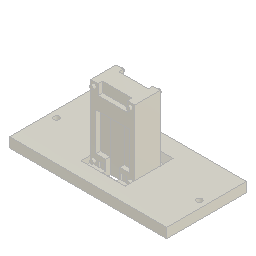
Nabu-SD-Backplate (Autodesk Fusion 360 design; units mm, degrees)
Autodesk Fusion 360 part; units mm, degrees
sketch "Sketch1" plane through (0, 0, 0) normal (0, 0, 1) x (1, 0, 0)
  line L0 (-42.75, -21.675) -> (42.75, -21.675)
  line L1 (42.75, -21.675) -> (42.75, 21.675)
  line L2 (42.75, 21.675) -> (-42.75, 21.675)
  line L3 (-42.75, 21.675) -> (-42.75, -21.675)
  line L4 (-35.5, -20) -> (35.5, -20)
  line L5 (35.5, 20) -> (35.5, -20)
  line L6 (35.5, 20) -> (-35.5, 20)
  line L7 (-35.5, -20) -> (-35.5, 20)
  line L8 (-38.85, 0) -> (38.85, 0) construction
  circle A0 centre (38.85, 0) radius 1.5
  circle A1 centre (-38.85, 0) radius 1.5
  line L9 (0, 20) -> (0, 11) construction
  line L10 (0, 11) -> (0, 5) construction
  line L11 (0, 5) -> (0, -4) construction
  line L12 (0, -4) -> (0, -10) construction
  line L13 (0, -10) -> (0, -20) construction
  circle A2 centre (0, 8) radius 0.9 construction
  circle A3 centre (0, -7) radius 1.325 construction
  circle A4 centre (0, 6.3) radius 0.8 construction
  circle A5 centre (0, -9.125) radius 0.8 construction
  line L14 (-6.875, 8.9) -> (6.875, 8.9)
  line L15 (6.875, 8.9) -> (6.875, 7.1)
  line L16 (6.875, 7.1) -> (-6.875, 7.1)
  line L17 (-6.875, 7.1) -> (-6.875, 8.9)
  line L18 (-3.8, -5.675) -> (3.8, -5.675)
  line L19 (3.8, -5.675) -> (3.8, -8.325)
  line L20 (3.8, -8.325) -> (-3.8, -8.325)
  line L21 (-3.8, -8.325) -> (-3.8, -5.675)
  line L22 (-12, 7.1) -> (12, 7.1)
  line L23 (12, 7.1) -> (12, 5.5)
  line L24 (12, 5.5) -> (-12, 5.5)
  line L25 (-12, 5.5) -> (-12, 7.1)
  line L26 (-12, -8.325) -> (12, -8.325)
  line L27 (12, -8.325) -> (12, -9.925)
  line L28 (12, -9.925) -> (-12, -9.925)
  line L29 (-12, -9.925) -> (-12, -8.325)
  line L30 (-7.5, -7.325) -> (7.5, -7.325) construction
  line L31 (-7.5, -8.325) -> (-7.5, -7.325)
  line L32 (-7.5, -7.825) -> (-4.5, -7.825) construction
  line L33 (7.5, -7.325) -> (7.5, -8.325)
  line L34 (7.5, -7.825) -> (4.5, -7.825) construction
  line L35 (-4.5, -8.325) -> (-4.5, -7.325)
  line L36 (4.5, -8.325) -> (4.5, -7.325)
  line L37 (-7.5, -7.325) -> (-4.5, -7.325)
  line L38 (4.5, -7.325) -> (7.5, -7.325)
  line L39 (-12, -8.325) -> (-12, 5.5)
  line L40 (12, -8.325) -> (12, 5.5)
  line L41 (6.875, 8.9) -> (12, 8.9)
  line L42 (12, 8.9) -> (12, 7.1)
  line L43 (-6.875, 8.9) -> (-12, 8.9)
  line L44 (-12, 8.9) -> (-12, 7.1)
  line L45 (-9.2, -8.325) -> (-9.2, -5.825)
  line L46 (-12, -5.825) -> (-9.2, -5.825)
  line L47 (12, -5.825) -> (9.2, -5.825)
  line L48 (9.2, -8.325) -> (9.2, -5.825)
  line L49 (-12, 3) -> (-8, 3)
  line L50 (-8, 5.5) -> (-8, 3)
  line L51 (12, 3) -> (8, 3)
  line L52 (8, 5.5) -> (8, 3)
  line L53 (8, 3) -> (-8, 3)
  line L54 (-8, -8.325) -> (-8, -5.825)
  line L55 (8, -8.325) -> (8, -5.825)
  line L56 (9.2, -5.825) -> (-9.2, -5.825)
  point P0 (42.75, 0)
  point P1 (0, -21.675)
  point P2 (0, -20)
  point P3 (35.5, 0)
  point P4 (0, -5.675)
  point P5 (3.8, -7)
  point P6 (0, 8.9)
  point P7 (6.875, 8)
  point P8 (0, -9.925)
  point P9 (12, -9.125)
  point P10 (12, 6.3)
  point P11 (0, 5.5)
  point P12 (0, -7.325)
  dimension "d1" = 85.5
  dimension "d2" = 43.35
  dimension "d3" = 71
  dimension "d4" = 40
  dimension "d5" = 77.7
  dimension "d6" = 3
  dimension "d8" = 9
  dimension "d9" = 6
  dimension "d10" = 9
  dimension "d11" = 6
  dimension "d12" = 10
  dimension "d13" = 1.8
  dimension "d14" = 2.65
  dimension "d15" = 1.6
  dimension "d16" = 1.6
  dimension "d17" = 13.75
  dimension "d18" = 1.8
  dimension "d19" = 7.6
  dimension "d20" = 2.65
  dimension "d21" = 24
  dimension "d22" = 1.6
  dimension "d23" = 24
  dimension "d24" = 1.6
  dimension "d25" = 15
  dimension "d26" = 1
  dimension "d27" = 3
  dimension "d28" = 3
  dimension "d47" = 2.5
  dimension "d48" = 2.8
  dimension "d49" = 2.8
  dimension "d50" = 2.5
  dimension "d54" = 4
  dimension "d55" = 2.5
  dimension "d56" = 4
  dimension "d57" = 2.5
  dimension "d58" = 4
  dimension "d59" = 4
  constraint horizontal L0
  constraint perpendicular L0 L1
  constraint midpoint L1 P0
  constraint midpoint L0 P1
  constraint perpendicular L1 L2
  constraint equal L0 L2
  constraint perpendicular L2 L3
  constraint equal L1 L3
  constraint horizontal L4
  constraint vertical L5
  constraint midpoint L4 P2
  constraint midpoint L5 P3
  constraint horizontal P0 P3
  constraint vertical P1 P2
  constraint coincident L4.end L5.end
  constraint vertical P1 origin
  constraint horizontal P0 origin
  constraint perpendicular L5 L6
  constraint perpendicular L4 L7
  constraint equal L4 L6
  constraint equal L5 L7
  constraint horizontal L8
  constraint midpoint L8 origin
  constraint coincident L8.end A0.centre
  constraint coincident L8.start A1.centre
  constraint equal A0 A1
  constraint vertical L9
  constraint parallel L9 L10
  constraint parallel L10 L11
  constraint parallel L11 L12
  constraint parallel L12 L13
  constraint horizontal L5.start L9.start
  constraint midpoint L10 A2.centre
  constraint midpoint L12 A3.centre
  constraint tangent A2 A4
  constraint tangent A3 A5
  constraint horizontal L14
  constraint vertical L15
  constraint horizontal L16
  constraint vertical L17
  constraint horizontal L18
  constraint vertical L19
  constraint horizontal L20
  constraint vertical L21
  constraint midpoint L18 P4
  constraint midpoint L19 P5
  constraint midpoint L14 P6
  constraint midpoint L15 P7
  constraint horizontal A2.centre P7
  constraint horizontal A3.centre P5
  constraint vertical P4 P6
  constraint vertical origin P4
  constraint horizontal L22
  constraint vertical L23
  constraint horizontal L24
  constraint vertical L25
  constraint horizontal L26
  constraint vertical L27
  constraint horizontal L28
  constraint vertical L29
  constraint midpoint L28 P8
  constraint midpoint L27 P9
  constraint midpoint L23 P10
  constraint midpoint L24 P11
  constraint horizontal A5.centre P9
  constraint horizontal A4.centre P10
  constraint coincident origin L11
  constraint vertical P8 P11
  constraint vertical origin P8
  constraint horizontal L30
  constraint midpoint L30 P12
  constraint vertical origin P12
  constraint perpendicular L24 L31
  constraint coincident L26 L31.start
  constraint coincident L30.start L31.end
  constraint midpoint L31 L32.start
  constraint perpendicular L31 L32
  constraint coincident L26 L33.end
  constraint perpendicular L26 L33
  constraint midpoint L33 L34.start
  constraint perpendicular L33 L34
  constraint coincident L26 L35.start
  constraint coincident L30 L35.end
  constraint perpendicular L30 L35
  constraint coincident L26 L36.start
  constraint coincident L30 L36.end
  constraint perpendicular L30 L36
  constraint perpendicular L35 L37
  constraint perpendicular L33 L38
  constraint perpendicular L15 L41
  constraint perpendicular L22 L42
  constraint perpendicular L17 L43
  constraint vertical L44
  constraint coincident L26 L45.start
  constraint perpendicular L26 L45
  constraint coincident L39 L46.start
  constraint perpendicular L39 L46
  constraint coincident L45.end L46.end
  constraint coincident L40 L47.start
  constraint perpendicular L40 L47
  constraint coincident L26 L48.start
  constraint perpendicular L26 L48
  constraint coincident L47.end L48.end
  constraint coincident L39 L49.start
  constraint perpendicular L39 L49
  constraint coincident L24 L50.start
  constraint perpendicular L49 L50
  constraint coincident L49.end L50.end
  constraint coincident L40 L51.start
  constraint perpendicular L40 L51
  constraint coincident L24 L52.start
  constraint perpendicular L24 L52
  constraint coincident L51.end L52.end
  constraint coincident L26 L54.start
  constraint coincident L26 L55.start
  measures "d1" distance of L0.start L0.end
  measures "d2" distance of L0.end L1.end
  measures "d3" distance of L4.start L4.end
  measures "d4" distance of L5.start L4.end
  measures "d5" distance of L8.start L8.end
  measures "d6" diameter of A0
  measures "d8" distance of L9.start L9.end
  measures "d9" distance of L9.end L10.end
  measures "d10" distance of L10.end L11.end
  measures "d11" distance of L11.end L12.end
  measures "d12" distance of L12.end P2
  measures "d13" diameter of A2
  measures "d14" diameter of A3
  measures "d15" diameter of A4
  measures "d16" diameter of A5
  measures "d17" distance of L14.start L14.end
  measures "d18" distance of L14.start L16.end
  measures "d19" distance of L18.start L18.end
  measures "d20" distance of L18.start L20.end
  measures "d21" distance of L22.start L22.end
  measures "d22" distance of L22.start L24.end
  measures "d23" distance of L26.start L26.end
  measures "d24" distance of L26.start L28.end
  measures "d25" distance of L30.start L30.end
  measures "d26" distance of L31.start L30.start
  measures "d27" distance of L32.start L32.end
  measures "d28" distance of L34.start L34.end
  measures "d47" distance of L45.start L45.end
  measures "d48" distance of L46.start L45.end
  measures "d49" distance of L47.start L47.end
  measures "d50" distance of L48.start L47.end
  measures "d54" distance of L49.start L49.end
  measures "d55" distance of L50.start L49.end
  measures "d56" distance of L51.start L51.end
  measures "d57" distance of L52.start L51.end
  measures "d58" distance of L26.start L54.start
  measures "d59" distance of L26.end L55.start
extrude "Extrude1" add sketch "Sketch1" along normal blind 1 contours L4 L5 L6 L7 | L17 L22 L43 L44 | L15 L22 L41 L42 | L16 L22 L23 L24 L25 | L24 L39 L49 L50 | L24 L40 L51 L52 | L24 L50 L52 L53 | L18 L19 L21 L39 L40 L46 L47 L49 L51 L53 L56 | L26 L39 L45 L46 | L26 L40 L47 L48 | L20 L26 L27 L28 L29 | L26 L45 L54 L56 | L26 L48 L55 L56 | L21 L26 L31 L35 L37 L54 L56 | L19 L26 L33 L36 L38 L55 L56
extrude "Extrude2" add sketch "Sketch1" along normal blind 2 from surface at 1 contours L0 L1 L2 L3 | L4 L5 L6 L7 | L17 L22 L43 L44 | L15 L22 L41 L42 | L16 L22 L23 L24 L25 | L24 L39 L49 L50 | L24 L40 L51 L52 | L24 L50 L52 L53 | L18 L19 L21 L39 L40 L46 L47 L49 L51 L53 L56 | L26 L39 L45 L46 | L26 L40 L47 L48 | L20 L26 L27 L28 L29 | L26 L45 L54 L56 | L26 L48 L55 L56 | L21 L26 L31 L35 L37 L54 L56 | L19 L26 L33 L36 L38 L55 L56
extrude "Extrude3" add sketch "Sketch1" along normal blind 3.35 from surface at 3 contours L0 L1 L2 L3 | L4 L5 L6 L7
draft "Draft1" angle -30 neutral plane through (0, 0, 0) pull (0, 0, -1) 3 faces at (-2.2917, 8.9, 5.2333) (4, -9.925, 4.1167) (1.2667, -8.325, 1)
extrude "Extrude4" add sketch "Sketch1" along normal blind 3 from surface at 3 contours L24 L39 L49 L50 | L24 L40 L51 L52 | L24 L50 L52 L53 | L18 L19 L21 L39 L40 L46 L47 L49 L51 L53 L56 | L26 L39 L45 L46 | L26 L40 L47 L48 | L26 L45 L54 L56 | L26 L48 L55 L56 | L21 L26 L31 L35 L37 L54 L56 | L19 L26 L33 L36 L38 L55 L56
extrude "Extrude5" add sketch "Sketch1" along normal blind 2.5 from surface at 6 contours L24 L39 L49 L50 | L24 L40 L51 L52 | L24 L50 L52 L53 | L18 L19 L21 L39 L40 L46 L47 L49 L51 L53 L56 | L26 L39 L45 L46 | L26 L40 L47 L48 | L26 L45 L54 L56 | L26 L48 L55 L56 | L21 L26 L31 L35 L37 L54 L56 | L19 L26 L33 L36 L38 L55 L56 | L26 L31 L35 L37 | L26 L33 L36 L38
ref_plane "WorkPlane1" through (-7.9, -8.325, 5.75) normal (0, -1, 0) x (1, 0, 0)
ref_plane "WorkPlane2" through (0, 5.5, 5.75) normal (0, 1, 0) x (-1, 0, 0)
extrude "Extrude6" add sketch "Sketch1" along normal blind 20.5 from surface at 6 contours L24 L39 L49 L50 | L24 L40 L51 L52 | L24 L50 L52 L53 | L18 L19 L21 L39 L40 L46 L47 L49 L51 L53 L56 | L26 L39 L45 L46 | L26 L40 L47 L48
extrude "Extrude7" add sketch "Sketch1" along normal blind 10 from surface at 26.5 contours L24 L39 L49 L50 | L24 L40 L51 L52 | L24 L50 L52 L53 | L18 L19 L21 L39 L40 L46 L47 L49 L51 L53 L56 | L26 L39 L45 L46 | L26 L40 L47 L48 | L26 L45 L54 L56 | L26 L48 L55 L56 | L21 L26 L31 L35 L37 L54 L56 | L19 L26 L33 L36 L38 L55 L56 | L19 L20 L21 L26 L56 | L18 L19 L21 L56 | L26 L31 L35 L37 | L26 L33 L36 L38
draft "Draft2" angle 45 neutral plane through (-3.8, -5.675, 6) pull (0, -1, 0) 1 faces at (1.2667, -7.4917, 26.5)
extrude "Extrude8" add sketch "Sketch1" along normal blind 5.5 from surface at 36.5 contours L24 L39 L49 L50 | L24 L40 L51 L52 | L18 L19 L21 L39 L40 L46 L47 L49 L51 L53 L56 | L26 L39 L45 L46 | L26 L40 L47 L48 | L26 L45 L54 L56 | L26 L48 L55 L56 | L18 L19 L21 L56
sketch "Sketch2" plane through (0, -8.325, 0) normal (0, -1, 0) x (1, 0, 0)
  line L0 (12, 3) -> (12, 6.35)
  line L1 (12, 6.35) -> (12, 42)
  line L2 (12, 42) -> (8, 42)
  line L3 (8, 36.5) -> (-8, 36.5)
  line L4 (-8, 36.5) -> (-8, 42)
  line L5 (-8, 42) -> (-12, 42)
  line L6 (-12, 42) -> (-12, 6.35)
  line L7 (-12, 6.35) -> (-12, 3)
  line L8 (-12, 3) -> (-7.5, 3)
  line L9 (-7.5, 3) -> (-7.5, 6)
  line L10 (-7.5, 6) -> (-4.5, 6)
  line L11 (-4.5, 6) -> (-4.5, 3)
  line L12 (-4.5, 3) -> (-3.8, 3)
  line L13 (-3.8, 3) -> (-3.8, 8.5)
  line L14 (-3.8, 8.5) -> (-9.2, 8.5)
  line L15 (-9.2, 8.5) -> (-9.2, 29.15)
  line L16 (-9.2, 29.15) -> (9.2, 29.15)
  line L17 (9.2, 29.15) -> (9.2, 8.5)
  line L18 (9.2, 8.5) -> (3.8, 8.5)
  line L19 (3.8, 8.5) -> (3.8, 3)
  line L20 (3.8, 3) -> (4.5, 3)
  line L21 (4.5, 3) -> (4.5, 6)
  line L22 (4.5, 6) -> (7.5, 6)
  line L23 (7.5, 6) -> (7.5, 3)
  line L24 (7.5, 3) -> (12, 3)
  line L25 (8, 42) -> (8, 36.5)
  line L26 (10, 3) -> (10, 42) construction
  line L27 (-10, 3) -> (-10, 42) construction
  line L28 (12, 5) -> (-12, 5) construction
  line L29 (12, 40) -> (-12, 40) construction
  circle A0 centre (10, 5) radius 1
  circle A1 centre (-10, 5) radius 1
  circle A2 centre (10, 40) radius 1
  circle A3 centre (-10, 40) radius 1
  dimension "d68" = 2
  dimension "d69" = 2
  dimension "d70" = 2
  dimension "d71" = 2
  dimension "d74" = 2
  constraint coincident L24 L26.start
  constraint coincident L2 L26.end
  constraint perpendicular L2 L26
  constraint coincident L8 L27.start
  constraint perpendicular L8 L27
  constraint coincident L0 L28.start
  constraint coincident L7 L28.end
  constraint perpendicular L7 L28
  constraint coincident L1 L29.start
  constraint perpendicular L26 L29
  constraint coincident L28 A0.centre
  constraint coincident L26 A0.centre
  constraint coincident L28 A1.centre
  constraint coincident L27 A1.centre
  constraint coincident L29 A2.centre
  constraint coincident L26 A2.centre
  constraint coincident L29 A3.centre
  constraint coincident L27 A3.centre
  constraint equal A2 A3
  constraint equal A0 A2
  constraint equal A0 A1
  measures "d68" distance of L26.end L29
  measures "d69" distance of L1 L26
  measures "d70" distance of L27 L29.end
  measures "d71" distance of L26.start L28
  measures "d74" diameter of A2
extrude "Extrude9" add sketch "Sketch2" along normal mid plane 17.025 from surface at -6.9125 contours A0 | A1 | A2 | A3
equation "d37 = 30.00 °"
equation "d38 = 0.00 °"
equation "d63 = 45.00 °"
equation "d64 = 0.00 °"
